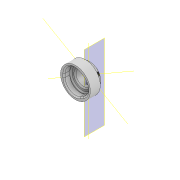
# Autodesk Inventor part: 30_Linear_Stage_NEMA11_baseholder_bayonetmount_objective_RMS_v0
Saved by Autodesk Inventor 2022 (Build 260153000, 153)
## iProperties
Created: 2023-02-17
Part Number: 30_Linear_Stage_NEMA11_baseholder_bayonetmount_objective_RMS_v0
Material: Generisch
Document SubType Name: Modeling
Designer: diederichbenedict
Density: 1 g/cm^3
Appearance: Vorgabe
Vendor: openUC2
Author: diederichbenedict
Autodesk Inventor part; units mm, degrees
ref_plane "YZ Plane" through (0, 0, 0) normal (1, 0, 0) x (0, 1, 0)
ref_plane "XZ Plane" through (0, 0, 0) normal (0, 1, 0) x (-1, 0, 0)
ref_plane "XY Plane" through (0, 0, 0) normal (0, 0, 1) x (1, 0, 0)
ref_plane "Arbeitsebene1" through (15, 0, 0) normal (-1, 0, 0) x (0, 1, 0)
sketch "Skizze1" plane through (15, 0, 0) normal (-1, 0, 0) x (0, 1, 0)
  line L0 (32.603074, 0.5) -> (30.723689, 0.5)
  line L1 (30.723689, 4.25) -> (32.603074, 4.25)
  line L2 (30.723689, 0.5) -> (30.723689, 4.25)
  line L3 (32.603074, 0.5) -> (30.723689, 0.5)
  line L4 (30.723689, 4.7) -> (32.603074, 4.7)
  line L5 (30.723689, 0.5) -> (30.723689, 4.25)
  line L6 (30, 0.5) -> (32, 0.5)
  line L7 (30, 0.55) -> (30, 0.5)
  line L8 (32, 0.5) -> (32, 0.55)
  line L9 (32, 0.5) -> (32, 16.1)
  line L10 (52, 0.5) -> (52, 16.1)
  line L11 (42, 19.32) -> (42, -3.22)
  line L12 (32.603074, 0.5) -> (29, 0.5)
  line L13 (29, 0.5) -> (29, -2.5)
  line L14 (29, -2.5) -> (35.603074, -2.5)
  line L15 (35.603074, -2.5) -> (35.603074, 5.25)
  line L16 (35.603074, 5.25) -> (34.103074, 5.25)
  line L17 (32.603074, 0.5) -> (32.603074, 0.2)
  line L18 (32.603074, 0.2) -> (29, 0.2)
  line L19 (32, 0.55) -> (30, 0.55)
  line L20 (32.103074, 0.5) -> (32.04123, 0.2)
  line L21 (29, -2.5) -> (33, -2.5)
  line L22 (33, -2.5) -> (33, -8.5)
  line L23 (33, -8.5) -> (29, -8.5)
  line L24 (29, -8.5) -> (29, -2.5)
  line L25 (34.103074, 5.25) -> (32.306983, 3.917608)
  line L26 (32.306983, 3.917608) -> (32.103074, 0.5)
  point P0 (0, 0)
  point P1 (33, -2.5)
  point P2 (30.723689, 0.55)
  point P3 (32, 4.25)
  dimension "d1" = 3
  dimension "d3" = 1
  dimension "d11" = 0.5
  dimension "d13" = 13
  dimension "d14" = 6
  dimension "d15" = 9
  dimension "d37" = 0.3
  dimension "d38" = 6.39693
  constraints: 34 end point, 5 perpendicular, 4 vertical, 3 point on line, 2 parallel, 1 coincident, 1 collinear, 1 horizontal, 5 other
  measures "d1" distance between parallel lines of L12 L14
  measures "d3" distance between parallel lines of L1 L16
  measures "d11" distance of L0.start L20.start
  measures "d13" distance between parallel lines of L13 L11
  measures "d14" distance of L21.end L22.end
  measures "d15" distance between parallel lines of L11 L22
  measures "d37" distance between parallel lines of L18 L0
  measures "d38" distance between parallel lines of L15 L11
revolve "Umdrehung1" add sketch "Skizze1" angle 360 about axis through (15, 42, -19.32) along (0, 0, 1) contours L17 L18 L20 L0 | L0 L26 L25 L16 L15 L14 L13 L18 L17 | L14 L22 L23 L24
sketch "Skizze2" plane through (0, 0, 0) normal (0, 1, 0) x (-1, 0, 0)
  spline S0 degree 3 poles (-15, -4.25) (-12.130398, -4.478356) (-9.273158, -4.706711) (-7.110863, -4.935067) (-6.855445, -4.962041) (-6.609475, -4.989015) (-6.373835, -5.01599) knots 0 0 0 0 0.71740042 0.71740042 0.71740042 0.80214247 0.80214247 0.80214247 0.80214247
  spline S1 degree 3 poles (-14.501577, -1.089675) (-11.631419, -1.318272) (-8.818268, -1.546869) (-6.735497, -1.775466) (-6.205432, -1.833644) (-5.721517, -1.891822) (-5.291796, -1.95) knots 0.04154724 0.04154724 0.04154724 0.04154724 0.75970637 0.75970637 0.75970637 0.9424778 0.9424778 0.9424778 0.9424778
  circle A0 centre (-15, -2.813821) radius 1.4
  line L0 (-15, 1.004794) -> (-15, -6.028763)
  point P0 (0, 0)
  dimension "d5" = 2.8
  constraints: 1 centre point, 1 point on line
  measures "d5" diameter of A0
extrude "Extrusion1" cut sketch "Skizze2" along normal up to surface
pattern_circular "Runde Anordnung1" count 3 over 360 about axis through (15, 42, 4.15) along (0, 0, -1) of "Extrusion1"
sketch "Skizze7" plane through (15, 42, 8.5) normal (0, 0, 1) x (1, 0, 0)
  circle A0 centre (0, 0) radius 13
  line L0 (6.3, -7.794229) -> (3.6, -9.353074)
  line L1 (-9.9, -1.558846) -> (-9.9, 1.558846)
  line L2 (3.6, 9.353074) -> (6.3, 7.794229)
  circle A1 centre (0, 0) radius 9.9
  line L3 (-15, 28.976764) -> (-15, -53.829461)
  arc A2 (6.3, -7.794229) -> (6.3, 7.794229) centre (1.8, 0) ccw
  arc A3 (-9.9, -1.558846) -> (3.6, -9.353074) centre (-0.9, -1.558846) ccw
  arc A4 (3.6, 9.353074) -> (-9.9, 1.558846) centre (-0.9, 1.558846) ccw
  point P0 (-15, -42)
  point P1 (19.8, 0)
  point P2 (-9.9, -17.147303)
  point P3 (-9.9, 17.147303)
  dimension "d39" = 19.8
  dimension "d40" = 9
  constraints: 7 tangent, 6 end point, 6 point on circle, 6 point on line, 4 centre point, 2 equal radius, 1 coincident, 1 parallel, 7 other
  measures "d39" diameter of A1
  measures "d40" radius of A2
extrude "Extrusion5" cut sketch "Skizze7" against normal blind 5 contours L0 A1 L2 A2 | L0 A3 L1 A1 | A1 | L1 A4 L2 A1
chamfer "Fase4" distance 1 angle 45 8 edges at (9.6, 51.3531, 8.5) (19.95, 50.5737, 8.5) (25.8, 42, 8.5) (19.95, 33.4263, 8.5) (9.6, 32.6469, 8.5) (5.1, 42, 8.5) (15, 51, 3.5) (15, 48.3969, 2.5)
